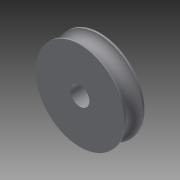
# Autodesk Inventor part: CarAxelGear
Saved by Autodesk Inventor 2015 (Build 190159000, 159)
## iProperties
Created: 2016-03-26
Part Number: CarAxelGear
Material: Generic
Document SubType Name: Modeling
Designer: Lee
Density: 1 g/cm^3
Appearance: Default
Author: Lee
Autodesk Inventor part; units mm, degrees
ref_plane "YZ Plane" through (0, 0, 0) normal (1, 0, 0) x (0, 1, 0)
ref_plane "XZ Plane" through (0, 0, 0) normal (0, 1, 0) x (-1, 0, 0)
ref_plane "XY Plane" through (0, 0, 0) normal (0, 0, 1) x (1, 0, 0)
sketch "Sketch1" plane through (0, 0, 0) normal (0, 0, 1) x (1, 0, 0)
  circle A0 centre (0, 0) radius 2.032
  circle A1 centre (0, 0) radius 9.525
  dimension "d0" = 4.064
  dimension "d1" = 19.05
  constraints: 2 centre point, 2 coincident
  measures "d0" diameter of A0
  measures "d1" diameter of A1
extrude "Extrusion1" add sketch "Sketch1" along normal blind 4.318
sketch "Sketch2" plane through (0, 0, 0) normal (0, 1, 0) x (-1, 0, 0)
  line L0 (9.525, 0) -> (9.525, 4.318) projected
  line L1 (9.525, 4.318) -> (-9.525, 4.318) projected
  line L2 (-9.525, 0) -> (9.525, 0) projected
  line L3 (9.525, 4.318) -> (7.8277, 2.6207)
  line L4 (9.525, 4.318) -> (14.8463, 4.318) construction
  line L5 (9.525, 0) -> (7.8277, 2.6207)
  arc A0 (9.525, 3.918) -> (9.525, 0.4) centre (9.525, 2.159) ccw
  line L6 (0, -0.8636) -> (0, 5.1816) projected
  point P0 (0, 0)
  dimension "d4" = 135
  dimension "d5" = 0.4
  dimension "d6" = 0.4
  constraints: 6 end point, 3 point on circle, 2 point on line, 1 centre point, 1 coincident, 1 horizontal
  measures "d4" angle of L3 L4
  measures "d5" distance from line of L1 A0.start
  measures "d6" distance from line of L2 A0.end
revolve "Revolution1" cut sketch "Sketch2" angle 360 about axis through (0, 0, -10) along (0, 0, 1) contours A0 L5 L3 L0 | A0 L5 | A0 L3
body "Solid1"
